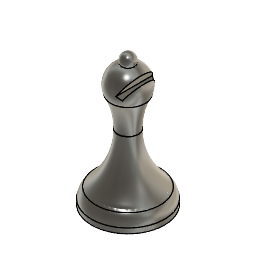
fou (Autodesk Fusion 360 design; units mm, degrees)
part number: 2026-06-29-12-18-11-648
Autodesk Fusion 360 part; units mm, degrees
sketch "Esquisse1" plane through (0, 0, 0) normal (0, 1, 0) x (1, 0, 0)
  line L0 (0, 0) -> (0, -38)
  line L1 (0, 0) -> (10.5, 0)
  circle A0 centre (0, -36) radius 2
  circle A1 centre (0, -29.9715) radius 5.5
  line L2 (3, -8) -> (3, -25.3617)
  line L3 (0, 0) -> (4.1, 0)
  line L4 (4.1, 0) -> (4.1, -3.2)
  line L5 (4.1, -3.2) -> (0, -3.2)
  line L6 (0, -3.2) -> (0, 0)
  line L7 (10.5, 0) -> (10.5, -3.2951)
  line L8 (10.5, -3.2951) -> (3, -8)
  dimension "d1" = 38
  dimension "d2" = 10.5
  dimension "d3" = 11
  dimension "d4" = 3
  dimension "d5" = 4.1
  dimension "d6" = 3.2
  dimension "d7" = 8
  constraint coincident L0.start L1.start
  constraint vertical L0
  constraint perpendicular L0 L1
  constraint coincident L0 A0.centre
  constraint coincident L0.end A0
  constraint coincident L0 A1.centre
  constraint coincident A1 L2.end
  constraint vertical L2
  constraint horizontal L3
  constraint vertical L4
  constraint horizontal L5
  constraint vertical L6
  constraint perpendicular L1 L7
  measures "d1" distance of L0.start L0.end
  measures "d2" distance of L0.start L1.end
  measures "d3" diameter of A1
  measures "d4" distance of L0 L2
  measures "d5" distance of L4.end L5.end
  measures "d6" distance of L3.end L4.end
  measures "d7" distance of L1 L2.start
revolve "Révolution1" add sketch "Esquisse1" angle 360 about axis through (0, 0, 0) along (0, 0, 1) contours L0 L1 A1 L2 L4 L5 L7 L8 | L0 A0 A1 | L0 A0 A1 | L0 A0 A1 picked at (0.2635, -27.6667) picked at (0.3925, -34.9963) picked at (0.5657, -36.197)
fillet "Congé1" radius 20 1 faces at (2.9851, -0.2987, 13.7872)
sketch "Esquisse2" plane through (0, 0, 0) normal (0, 1, 0) x (1, 0, 0)
  line L0 (3.9133, -34.1386) -> (1.7339, -30.3193)
  line L1 (1.7339, -30.3193) -> (3.0047, -29.5942)
  line L2 (3.0047, -29.5942) -> (5.4096, -33.3317)
  line L3 (5.4096, -33.3317) -> (3.9133, -34.1386)
  constraint perpendicular L0 L1
extrude "Extrusion1" cut sketch "Esquisse2" along normal blind 20 from surface at -10
fillet "Congé2" radius 4 1 edges at (-9.7894, -3.797, 3.2951)
